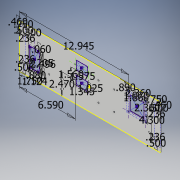
# Autodesk Inventor part: PDU_chassis_back
Saved by Autodesk Inventor 2017 (Build 210142000, 142)
## iProperties
Created: 2017-02-14
Part Number: PDU_chassis_back
Material: Generic
Document SubType Name: Modeling
Designer: Zara
Density: 1 g/cm^3
Appearance: Default
Author: Zara
Autodesk Inventor part; units mm, degrees
ref_plane "YZ Plane" through (0, 0, 0) normal (1, 0, 0) x (0, 1, 0)
ref_plane "XZ Plane" through (0, 0, 0) normal (0, 1, 0) x (-1, 0, 0)
ref_plane "XY Plane" through (0, 0, 0) normal (0, 0, 1) x (1, 0, 0)
sketch "Sketch1" plane through (0, 0, 0) normal (0, 0, 1) x (1, 0, 0)
  line L0 (-212.471, -66.294) -> (212.471, -66.294)
  line L1 (212.471, -66.294) -> (212.471, 66.294)
  line L2 (212.471, 66.294) -> (-212.471, 66.294)
  line L3 (-212.471, 66.294) -> (-212.471, -66.294)
  line L4 (-212.471, -66.294) -> (212.471, 66.294) construction
  line L5 (212.471, -66.294) -> (-212.471, 66.294) construction
  point P0 (0, 0)
  dimension "d0" = 424.942
  dimension "d1" = 132.588
  constraints: 12 end point, 2 midpoint, 2 parallel, 1 horizontal, 1 perpendicular
  measures "d0" distance of L1.end L2.end
  measures "d1" distance of L0.end L1.end
extrude "PDU back" add sketch "Sketch1" along normal blind 1.651
sketch "pwr entry" plane through (0, 0, 1.651) normal (0, 0, 1) x (1, 0, 0)
  line L0 (-180.7718, -40.259) -> (-155.2702, -40.259)
  line L1 (-153.7462, -38.735) -> (-153.7462, 14.224)
  line L2 (-155.2702, 15.748) -> (-180.7718, 15.748)
  line L3 (-182.2958, 14.224) -> (-182.2958, -38.735)
  line L4 (-182.2958, -40.259) -> (-153.7462, 15.748) construction
  line L5 (-153.7462, -40.259) -> (-182.2958, 15.748) construction
  line L6 (-168.021, 19.4437) -> (-168.021, -43.9547) construction
  line L7 (-212.471, 66.294) -> (-212.471, -66.294) projected
  line L8 (-212.471, -66.294) -> (212.471, -66.294) projected
  arc A0 (-153.7462, 14.224) -> (-155.2702, 15.748) centre (-155.2702, 14.224) ccw
  arc A1 (-180.7718, 15.748) -> (-182.2958, 14.224) centre (-180.7718, 14.224) ccw
  arc A2 (-182.2958, -38.735) -> (-180.7718, -40.259) centre (-180.7718, -38.735) ccw
  arc A3 (-155.2702, -40.259) -> (-153.7462, -38.735) centre (-155.2702, -38.735) ccw
  point P0 (0, 0)
  point P1 (-168.021, -12.2555)
  point P2 (-168.021, -12.2555)
  dimension "d4" = 56.007
  dimension "d5" = 28.5496
  dimension "d6" = 63.3984
  dimension "d7" = 44.45
  dimension "d8" = 22.3393
  dimension "d9" = 1.524
  constraints: 14 end point, 8 point on circle, 8 point on line, 8 tangent, 4 centre point, 4 midpoint, 3 equal radius, 2 coincident, 2 parallel, 1 horizontal, 1 perpendicular, 1 vertical
  measures "d4" distance of L5.start L4.end
  measures "d5" distance of L4.start L5.start
  measures "d6" distance of L6.end L6.start
  measures "d7" distance from line of L7 L6.end
  measures "d8" distance from line of point (-168.021, -43.955) L8
  measures "d9" radius of A0
extrude "pwr entry cutout" cut sketch "pwr entry" against normal through all
hole "pwr entry holes" at (-168.021, 19.4437, 1.651) at (-168.021, -43.9547, 1.651) direction (0, 0, -1) diameter 3.4544 end through all
sketch "IEC outlet" plane through (0, 0, 1.651) normal (0, 0, 1) x (1, 0, 0)
  line L0 (-42.164, -16.5735) -> (-8.001, -16.5735)
  line L1 (-8.001, -16.5735) -> (-8.001, 9.4615)
  line L2 (-8.001, 9.4615) -> (-42.164, 9.4615)
  line L3 (-42.164, 9.4615) -> (-42.164, -16.5735)
  line L4 (-42.164, -16.5735) -> (-8.001, 9.4615) construction
  line L5 (-8.001, -16.5735) -> (-42.164, 9.4615) construction
  line L6 (-45.085, -3.556) -> (-5.08, -3.556) construction
  line L7 (-212.471, 66.294) -> (-212.471, -66.294) projected
  line L8 (-212.471, -66.294) -> (212.471, -66.294) projected
  line L9 (-42.164, 23.0505) -> (-8.001, 23.0505)
  line L10 (-8.001, 23.0505) -> (-8.001, 49.0855)
  line L11 (-8.001, 49.0855) -> (-42.164, 49.0855)
  line L12 (-42.164, 49.0855) -> (-42.164, 23.0505)
  line L13 (-42.164, 23.0505) -> (-8.001, 49.0855) construction
  line L14 (-8.001, 23.0505) -> (-42.164, 49.0855) construction
  line L15 (-45.085, 36.068) -> (-5.08, 36.068) construction
  point P0 (-25.0825, -3.556)
  point P1 (-25.0825, -3.556)
  point P2 (-45.085, 36.068)
  point P3 (-5.08, 36.068)
  point P4 (-25.0825, 36.068)
  point P5 (-25.0825, 36.068)
  dimension "d19" = 26.035
  dimension "d20" = 34.163
  dimension "d22" = 40.005
  dimension "d23" = 167.386
  dimension "d24" = 62.738
  dimension "d129" = 39.624
  constraints: 28 end point, 6 midpoint, 4 coincident, 2 horizontal, 2 parallel, 1 collinear, 1 perpendicular, 1 vertical, 16 other
  measures "d19" distance of L0.end L1.end
  measures "d20" distance of L0.start L0.end
  measures "d22" distance of L6.end point (-45.085, -3.556)
  measures "d23" distance from line of L7 L6.start
  measures "d24" distance from line of L6.start L8
  measures "d129" distance of L0.start L9.start
hole "IEC holes" at (-5.08, -3.556, 1.651) at (-45.085, -3.556, 1.651) at (-45.085, 36.068, 1.651) at (-5.08, 36.068, 1.651) direction (0, 0, -1) diameter 3.4544 end through all
sketch "airflow" plane through (0, 0, 1.651) normal (0, 0, 1) x (1, 0, 0)
  line L0 (-212.471, 66.294) -> (-212.471, -66.294) projected
  line L1 (-212.471, -66.294) -> (212.471, -66.294) projected
  line L2 (111.379, -11.303) -> (171.323, -11.303) construction
  line L3 (171.323, -11.303) -> (171.323, 48.641) construction
  line L4 (171.323, 48.641) -> (111.379, 48.641) construction
  line L5 (111.379, 48.641) -> (111.379, -11.303) construction
  line L6 (111.379, -11.303) -> (171.323, 48.641) construction
  line L7 (171.323, -11.303) -> (111.379, 48.641) construction
  line L8 (116.332, -6.35) -> (166.37, -6.35) construction
  line L9 (166.37, -6.35) -> (166.37, 43.688) construction
  line L10 (166.37, 43.688) -> (116.332, 43.688) construction
  line L11 (116.332, 43.688) -> (116.332, -6.35) construction
  line L12 (116.332, -6.35) -> (166.37, 43.688) construction
  line L13 (166.37, -6.35) -> (116.332, 43.688) construction
  line L14 (120.269, -2.413) -> (162.433, -2.413)
  line L15 (162.433, -2.413) -> (162.433, 39.751)
  line L16 (162.433, 39.751) -> (120.269, 39.751)
  line L17 (120.269, 39.751) -> (120.269, -2.413)
  line L18 (120.269, -2.413) -> (162.433, 39.751) construction
  line L19 (162.433, -2.413) -> (120.269, 39.751) construction
  line L20 (212.471, 66.294) -> (-212.471, 66.294) projected
  point P0 (0, 0)
  point P1 (141.351, 18.669)
  point P2 (141.351, 18.669)
  dimension "d76" = 59.944
  dimension "d77" = 59.944
  dimension "d78" = 50.038
  dimension "d79" = 42.164
  dimension "d123" = 22.606
  dimension "d153" = 328.803
  constraints: 36 end point, 8 midpoint, 6 parallel, 4 coincident, 3 horizontal, 3 perpendicular, 2 point on line
  measures "d76" distance of L3.end L4.end
  measures "d77" distance of L2.end L3.end
  measures "d78" distance of L9.end L10.end
  measures "d79" distance of L15.end L16.end
  measures "d123" distance from line of L20 point (116.332, 43.688)
  measures "d153" distance from line of L0 point (116.332, 43.688)
sketch "relay holes" plane through (0, 0, 0) normal (0, 0, -1) x (-1, 0, 0)
  circle A0 centre (5.08, 36.068) radius 1.7272 construction
  circle A1 centre (5.08, -3.556) radius 1.7272 construction
  line L0 (5.08, 36.068) -> (5.08, -3.556) construction
  circle A2 centre (45.085, 36.068) radius 1.7272 construction
  line L1 (84.9503, 23.1654) -> (84.9503, -54.0444) construction
  line L2 (-212.471, 66.294) -> (212.471, 66.294) projected
  line L3 (5.08, 36.068) -> (5.08, -3.9037) construction
  line L4 (153.7462, 14.224) -> (153.7462, -38.735) projected
  line L5 (75.5142, -29.21) -> (123.2662, -29.21) construction
  point P0 (-25.527, -29.21)
  point P1 (-25.4, 29.21)
  point P2 (-73.152, 29.21)
  point P3 (-73.152, -29.21)
  point P4 (-25.4, -29.21)
  dimension "d138" = 47.752
  dimension "d139" = 37.084
  dimension "d143" = 58.42
  dimension "d148" = 47.752
  dimension "d149" = 95.504
  dimension "d150" = 30.48
  dimension "d152" = 30.48
  constraints: 8 end point, 2 vertical, 1 horizontal, 1 point on line
  measures "d138" distance of point (-73.152, 29.21) point (-25.4, 29.21)
  measures "d139" distance from line of point (-25.4, 29.21) L2
  measures "d143" distance of point (-73.152, 29.21) point (-73.152, -29.21)
  measures "d148" distance of L5.end L5.start
  measures "d149" distance between parallel lines of L2 L5
  measures "d150" distance from line of L4 L5.end
  measures "d152" horizontal distance of L3.start point (-25.4, 29.21)
hole "Hole5" at (166.37, 43.688, 1.651) at (116.332, 43.688, 1.651) at (116.332, -6.35, 1.651) at (166.37, -6.35, 1.651) direction (0, 0, -1) diameter 5.1054 end through all
extrude "Extrusion6" cut sketch "airflow" against normal blind 25.4
sketch "bracket" plane through (0, 0, 1.651) normal (0, 0, 1) x (1, 0, 0)
  line L0 (212.471, -66.294) -> (212.471, 66.294) construction
  line L1 (212.471, 54.61) -> (193.421, 54.61) construction
  line L2 (193.421, 54.61) -> (193.421, -54.61) construction
  line L3 (193.421, -54.61) -> (212.471, -54.61) construction
  line L4 (212.471, -54.61) -> (212.471, 54.61) construction
  line L5 (212.471, 66.294) -> (-212.471, 66.294) construction
  line L6 (-212.471, 66.294) -> (-212.471, -66.294) construction
  line L7 (-212.471, 54.61) -> (-193.421, 54.61) construction
  line L8 (-193.421, 54.61) -> (-193.421, -54.61) construction
  line L9 (-193.421, -54.61) -> (-212.471, -54.61) construction
  line L10 (-212.471, -54.61) -> (-212.471, 54.61) construction
  point P0 (0, 0)
  point P1 (199.4154, 41.91)
  point P2 (199.4154, -41.91)
  point P3 (-199.4154, -41.91)
  point P4 (-199.4154, 41.91)
  dimension "d94" = 19.05
  dimension "d95" = 109.22
  dimension "d96" = 11.684
  dimension "d103" = 19.05
  dimension "d104" = 109.22
  dimension "d105" = 11.684
  dimension "d121" = 12.7
  dimension "d122" = 5.9944
  dimension "d161" = 12.7
  dimension "d162" = 12.7
  dimension "d163" = 5.9944
  dimension "d164" = 5.9944
  dimension "d165" = 12.7
  dimension "d166" = 5.9944
  constraints: 16 end point, 4 parallel, 2 horizontal, 2 perpendicular, 2 point on line
  measures "d94" distance of L1.start L1.end
  measures "d95" distance of L1.end L2.end
  measures "d96" distance between parallel lines of L5 L1
  measures "d103" distance of L7.start L7.end
  measures "d104" distance of L7.end L8.end
  measures "d105" distance between parallel lines of L5 L7
  measures "d121" distance from line of L1 point (199.415, 41.91)
  measures "d122" distance from line of L2 point (199.415, 41.91)
  measures "d161" distance from line of point (-199.415, 41.91) L7
  measures "d162" distance from line of point (-199.415, -41.91) L9
  measures "d163" distance from line of L8 point (-199.415, -41.91)
  measures "d164" distance from line of point (-199.415, 41.91) L8
  measures "d165" distance from line of point (199.415, -41.91) L3
  measures "d166" distance from line of L2 point (199.415, -41.91)
hole "bracket holes" at (-199.4154, 41.91, 1.651) at (-199.4154, -41.91, 1.651) at (199.4154, 41.91, 1.651) at (199.4154, -41.91, 1.651) direction (0, 0, -1) diameter 4.2926 end through all clearance for "Countersunk Flat Head Screw ISO 2009/7046" size "M4" standard "ISO"
extrude "Extrusion7" cut sketch "IEC outlet" against normal through all
fillet "Fillet3" radius 4.9784 8 edges at (-42.164, 49.0855, 0.8255) (-42.164, 23.0505, 0.8255) (-8.001, 23.0505, 0.8255) (-8.001, 49.0855, 0.8255) (-8.001, 9.4615, 0.8255) (-42.164, 9.4615, 0.8255) (-42.164, -16.5735, 0.8255) (-8.001, -16.5735, 0.8255)
hole "Hole8" at (25.4, 29.21, 0) at (73.152, 29.21, 0) at (73.152, -29.21, 0) at (25.527, -29.21, 0) at (-123.2662, -29.21, 0) at (-75.5142, -29.21, 0) direction (0, 0, 1) diameter 4.4958 end through all clearance for "Flat Head Machine Screw (82)" size "#8" standard "Ansi Unified Screw Threads"
body "Solid1"
